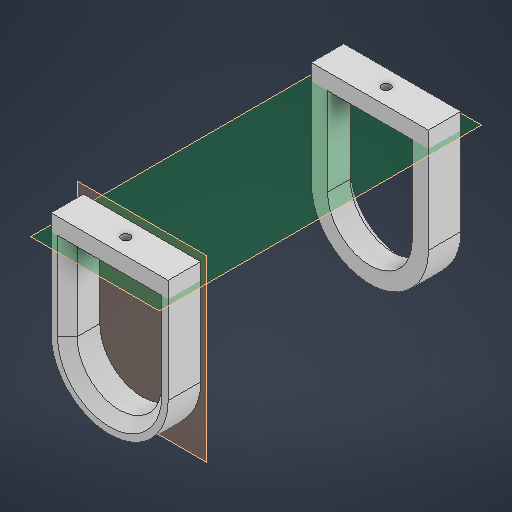
# Autodesk Inventor part: Payload Mount
Saved by Autodesk Inventor 2026.1 (Build 301233000, 233)
## iProperties
Created: 2026-03-28
Part Number: Payload Mount
Material: Generic
Document SubType Name: Modeling
Designer: elisa
Density: 1 g/cm^3
Appearance: Default
Author: elisa
Autodesk Inventor part; units mm, degrees
ref_plane "YZ Plane" through (0, 0, 0) normal (1, 0, 0) x (0, 1, 0)
ref_plane "XZ Plane" through (0, 0, 0) normal (0, 1, 0) x (-1, 0, 0)
ref_plane "XY Plane" through (0, 0, 0) normal (0, 0, 1) x (1, 0, 0)
sketch "Sketch1" plane through (0, 0, 0) normal (0, 0, 1) x (1, 0, 0)
  line L0 (170.0568, 0) -> (-170.0568, 0) construction
  line L1 (-170.0568, -123.761) -> (170.0568, -123.761) construction
  arc A0 (-26, -64) -> (26, -64) centre (0, -64) ccw
  line L2 (-36, 0) -> (-36, -64)
  arc A1 (-36, -64) -> (36, -64) centre (0, -64) ccw
  line L3 (36, -64) -> (36, 0)
  line L4 (-36, 0) -> (36, 0)
  line L5 (36, 0) -> (36, -10.8617)
  line L6 (26, -10) -> (-26, -10)
  line L7 (-36, -10) -> (-36, 0)
  line L8 (-26, -64) -> (-26, -10)
  line L9 (-26, 0) -> (-26, 0)
  line L10 (26, -64) -> (26, -10)
  line L11 (26, 0) -> (26, 0)
  point P0 (0, 0)
  point P1 (0, -90)
  point P2 (0, 0)
  point P3 (36, 0)
  dimension "d0" = 123.761
  dimension "d3" = 26
  dimension "d6" = 10
  dimension "d7" = 80
  constraints: 24 end point, 5 perpendicular, 5 point on circle, 5 point on line, 4 tangent, 3 horizontal, 2 centre point, 2 midpoint, 2 parallel, 1 coincident
  measures "d0" distance between parallel lines of L1 L0
  measures "d3" radius of A0
  measures "d6" distance between parallel lines of L6 L4
  measures "d7" distance from line of point (0, -90) L6
extrude "Rear Support" add sketch "Sketch1" along normal blind 20
ref_plane "Work Plane1" through (0, 0, 160) normal (0, 0, 1) x (1, 0, 0)
sketch "Sketch2" plane through (0, 0, 160) normal (0, 0, 1) x (1, 0, 0)
  line L0 (36, -64) -> (36, 0) projected
  line L1 (36, 0) -> (-36, 0) projected
  line L2 (-36, 0) -> (-36, -64) projected
  arc A0 (-36, -64) -> (36, -64) centre (0, -64) ccw projected
  line L3 (-26, -64) -> (-26, -10) projected
  line L4 (-26, -10) -> (26, -10) projected
  line L5 (26, -10) -> (26, -64) projected
  arc A1 (-26, -64) -> (26, -64) centre (0, -64) ccw projected
  point P0 (0, 0)
extrude "Front Support" add sketch "Sketch2" along normal blind 20
ref_plane "Work Plane2" through (-26, -10, 10) normal (0, -1, 0) x (1, 0, 0)
chamfer "Chamfer1" distance 6 angle 45 6 edges at (0, -90, 0) (-26, -37, 0) (26, -37, 0) (0, -90, 180) (-26, -37, 180) (26, -37, 180)
sketch "Sketch3" plane through (-26, -10, 10) normal (0, -1, 0) x (1, 0, 0)
  line L0 (62, 150) -> (62, 170) projected
  line L1 (62, 160) -> (-10, 160) construction
  line L2 (-10, 150) -> (-10, 170) projected
  line L3 (-6, 170) -> (58, 170) projected
  line L4 (26, 170) -> (26, 150) construction
  line L5 (0, 150) -> (52, 150) projected
  line L6 (62, -10) -> (62, 10) construction
  line L7 (62, 0) -> (-10, 0) construction
  line L8 (-10, -10) -> (-10, 10) construction
  line L9 (62, 10) -> (-10, 10) construction
  line L10 (26, 10) -> (26, -10) construction
  line L11 (-6, -10) -> (58, -10) construction
  circle A0 centre (26, 160) radius 4.5
  circle A1 centre (26, 0) radius 4.5
  dimension "d16" = 9
  constraints: 9 midpoint, 8 end point, 2 centre point, 1 equal radius, 1 perpendicular
  measures "d16" diameter of A0
extrude "Extrusion3" cut sketch "Sketch3" against normal blind 5
sketch "Sketch4" plane through (-36, 0, 160) normal (0, 1, 0) x (1, 0, 0)
  circle A0 centre (36, -10) radius 4.5 projected
  circle A1 centre (36, -10) radius 2.75
  circle A2 centre (36, 150) radius 4.5 projected
  circle A3 centre (36, 150) radius 2.75
  point P0 (36, 160)
  dimension "d19" = 5.5
  constraints: 2 centre point, 2 coincident
  measures "d19" diameter of A1
extrude "Extrusion4" cut sketch "Sketch4" against normal blind 10 contours A1 | A3
body "Solid1"
